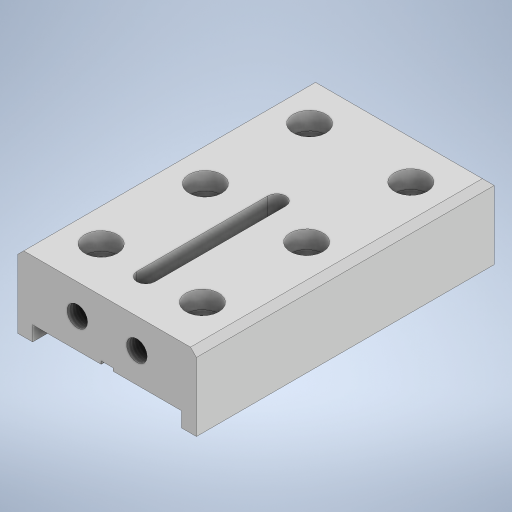
# Autodesk Inventor part: Part2
Saved by Autodesk Inventor 2024 (Build 280153000, 153)
## iProperties
Created: 2023-05-11
Part Number: Part2
Material: Generic
Document SubType Name: Modeling
Designer: Raj
Density: 1 g/cm^3
Appearance: Default
Author: Raj
Autodesk Inventor part; units mm, degrees
ref_plane "YZ Plane" through (0, 0, 0) normal (1, 0, 0) x (0, 1, 0)
ref_plane "XZ Plane" through (0, 0, 0) normal (0, 1, 0) x (-1, 0, 0)
ref_plane "XY Plane" through (0, 0, 0) normal (0, 0, 1) x (1, 0, 0)
sketch "Sketch3" plane through (0, 0, 0) normal (0, 0, 1) x (1, 0, 0)
  line L0 (0, 0) -> (60, 0)
  line L1 (60, 0) -> (60, 100)
  line L2 (60, 100) -> (0, 100)
  line L3 (0, 100) -> (0, 0)
  dimension "d6" = 60
  dimension "d7" = 100
  constraints: 8 end point, 2 parallel, 1 horizontal, 1 perpendicular
  measures "d6" distance of L2.end L1.end
  measures "d7" distance of L1.end L0.end
extrude "Extrusion1" add sketch "Sketch3" along normal blind 25
sketch "Sketch4" plane through (0, 0, 0) normal (0, -1, 0) x (1, 0, 0)
  line L0 (60, 0) -> (0, 0) projected
  line L1 (5, 0) -> (5, 5)
  line L2 (5, 5) -> (28, 5)
  line L3 (28, 5) -> (28, 6)
  line L4 (28, 6) -> (32, 6)
  line L5 (32, 6) -> (32, 5)
  line L6 (32, 5) -> (55, 5)
  line L7 (55, 5) -> (55, 0)
  line L8 (55, 0) -> (5, 0)
  line L9 (0, 0) -> (0, 25) projected
  dimension "d14" = 5
  dimension "d15" = 23
  dimension "d16" = 1
  dimension "d17" = 4
  dimension "d18" = 1
  dimension "d19" = 23
  dimension "d20" = 5
  dimension "d21" = 5
  constraints: 16 end point, 4 perpendicular, 4 point on line
  measures "d14" distance of L1.start L1.end
  measures "d15" distance of L1.end L2.end
  measures "d16" distance of L2.end L3.end
  measures "d17" distance of L3.end L4.end
  measures "d18" distance of L4.end L5.end
  measures "d19" distance of L5.end L6.end
  measures "d20" distance of L6.end L7.end
  measures "d21" distance between parallel lines of L9 L1
extrude "Extrusion2" cut sketch "Sketch4" against normal through all
sketch "Sketch5" plane through (0, 0, 25) normal (0, 0, 1) x (1, 0, 0)
  line L0 (0, 0) -> (60, 0) projected
  line L1 (0, 100) -> (0, 0) projected
  point P0 (47, 15)
  point P1 (47, 50)
  point P2 (47, 85)
  point P3 (13, 15)
  point P4 (13, 50)
  point P5 (13, 85)
  dimension "d24" = 15
  dimension "d25" = 47
  dimension "d28" = 35
  dimension "d31" = 34
  constraints: 1 horizontal, 1 vertical, 5 other
  measures "d24" distance from line of point (47, 15) L0
  measures "d25" distance from line of point (47, 15) L1
  measures "d28" distance of point (47, 15) point (47, 50)
  measures "d31" distance of point (47, 15) point (13, 15)
hole "Hole1" at (47, 15, 25) at (47, 50, 25) at (47, 85, 25) at (13, 15, 25) at (13, 50, 25) at (13, 85, 25) direction (0, 0, -1) diameter 6.4 end through all counterbore diameter 11 counterbore depth 6
sketch "Sketch6" plane through (0, 0, 25) normal (0, -1, 0) x (1, 0, 0)
  line L0 (0, 0) -> (60, 0) projected
  line L1 (0, -25) -> (0, 0) projected
  point P0 (20, -10)
  point P1 (40, -10)
  dimension "d41" = 10
  dimension "d42" = 10
  dimension "d43" = 20
  dimension "d44" = 20
  measures "d41" distance from line of point (20, -10) L0
  measures "d42" distance from line of L0 point (40, -10)
  measures "d43" distance of point (40, -10) point (20, -10)
  measures "d44" distance from line of L1 point (20, -10)
hole "Hole2" at (20, 0, 15) at (40, 0, 15) direction (0, 1, 0) diameter 6.917 depth 15 tip angle 118 thread size "M8x1" class "6H" standard "ISO Metric profile"
sketch "Sketch7" plane through (0, 0, 25) normal (0, 0, 1) x (1, 0, 0)
  line L0 (30, 13) -> (30, 57) construction
  line L1 (33, 13) -> (33, 57)
  line L2 (27, 57) -> (27, 13)
  arc A0 (27, 13) -> (33, 13) centre (30, 13) ccw
  arc A1 (33, 57) -> (27, 57) centre (30, 57) ccw
  line L3 (0, 0) -> (60, 0) projected
  point P0 (30, 35)
  dimension "d52" = 44
  dimension "d53" = 6
  dimension "d54" = 30
  dimension "d55" = 13
  constraints: 8 end point, 4 point on circle, 4 tangent, 2 centre point, 1 midpoint, 1 parallel, 1 vertical
  measures "d52" distance of L0.start L0.end
  measures "d53" diameter of A1
  measures "d54" horizontal distance of L3.start point (30, 35)
  measures "d55" distance from line of L3 L0.start
extrude "Extrusion3" cut sketch "Sketch7" against normal through all
chamfer "Chamfer2" distance 2 angle 45 3 edges at (0, 50, 25) (30, 100, 25) (60, 50, 25)
body "Solid1"
